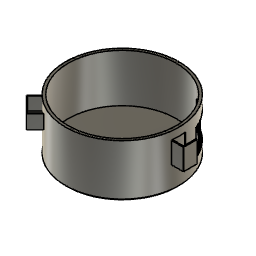
MedWise_shell v1 (Autodesk Fusion 360 design; units mm, degrees)
Autodesk Fusion 360 part; units mm, degrees
sketch "Sketch1" plane through (0, 0, 0) normal (0, 0, 1) x (1, 0, 0)
  circle A0 centre (0, 0) radius 65
  dimension "d1" = 130
  constraint coincident A0.centre origin
  measures "d1" diameter of A0
extrude "Extrude1" add sketch "Sketch1" along normal blind 60
hole "Hole1" at (0, 0, 60) direction (0, 0, -1) diameter 124 depth 55 tip angle 180
ref_plane "WorkPlane1" through (65, 0, 32.9588) normal (1, 0, 0) x (0, -1, 0)
ref_plane "WorkPlane2" through (77.5, 0, 32.9588) normal (1, 0, 0) x (0, -1, 0)
sketch "Sketch2" plane through (77.5, 0, 32.9588) normal (1, 0, 0) x (0, 1, 0)
  line L0 (-8, -8) -> (8, -8)
  line L1 (8, -8) -> (8, 18)
  line L2 (8, 18) -> (-8, 18)
  line L3 (-8, 18) -> (-8, -8)
  line L4 (-8, -8) -> (8, 18) construction
  line L5 (8, -8) -> (-8, 18) construction
  point P0 (0, 5)
  dimension "d9" = 16
  constraint horizontal L0
  constraint perpendicular L0 L1
  constraint parallel L0 L2
  constraint parallel L1 L3
  constraint coincident L4 P0
  constraint coincident L5 P0
  measures "d9" distance of L1.end L2.end
extrude "Extrude2" add sketch "Sketch2" along normal up to surface end surface at (64.677, -6.4719, 40)
extrude "Extrude3" add 1 faces at (77.5, -2.6667, 33.6254) along direction (1, 0, 0) blind 0.5
extrude "Extrude4" cut 1 faces at (73.6667, 0, 24.9588) along direction (0, 0, 1) blind 1
extrude "Extrude5" add 1 faces at (78, -2.6667, 42.6254) along direction (1, 0, 0) blind 0.2
shell "Shell1" thickness 1 removed faces 2 at (69.0705, 8, 34.2921) at (73.8, 0, 50.9588)
ref_plane "WorkPlane3" through (49.7929, 41.7812, 24.979) normal (0.766044, 0.642788, 0) x (0.642788, -0.766044, 0)
sketch "Sketch3" plane through (49.7929, 41.7812, 24.979) normal (0.766044, 0.642788, 0) x (0.642788, -0.766044, 0)
  line L0 (20, -20) -> (-20, -20)
  line L1 (-20, -20) -> (-20, 10)
  line L2 (-20, 10) -> (20, 10)
  line L3 (20, 10) -> (20, -20)
  line L4 (20, -20) -> (-20, 10) construction
  line L5 (-20, -20) -> (20, 10) construction
  point P0 (0, -5)
  dimension "d20" = 40
  constraint horizontal L0
  constraint perpendicular L0 L1
  constraint parallel L0 L2
  constraint parallel L1 L3
  constraint coincident L4 P0
  constraint coincident L5 P0
  measures "d20" distance of L1.end L2.end
extrude "Extrude6" cut sketch "Sketch3" against normal blind 20
fillet "Fillet1" radius 0.4 8 edges at (78.2, 0, 50.9588) (77.7, 8, 50.9588) (78.2, 8, 38.4588) (71.3529, 8, 25.9588) (78.2, 0, 25.9588) (78.2, -8, 38.4588) (71.3529, -8, 50.9588) (71.3529, -8, 25.9588)
fillet "Fillet2" radius 2 1 edges at (-60.6013, -23.505, 0)
ref_plane "WorkPlane4" through (49.7929, 41.7812, 24.979) normal (0.766044, 0.642788, 0) x (0.642788, -0.766044, 0)
ref_plane "WorkPlane5" through (-45.9619, -45.9619, 2.3267) normal (-0.707107, -0.707107, 0) x (-0.707107, 0.707107, 0)
ref_plane "WorkPlane6" through (-55.2958, -55.2958, 2.3267) normal (-0.707107, -0.707107, 0) x (-0.707107, 0.707107, 0)
sketch "Sketch4" plane through (-55.2958, -55.2958, 2.3267) normal (-0.707107, -0.707107, 0) x (-0.707107, 0.707107, 0)
  line L0 (13, -31.7116) -> (-13, -31.7116)
  line L1 (-13, -31.7116) -> (-13, -47.7116)
  line L2 (-13, -47.7116) -> (13, -47.7116)
  line L3 (13, -47.7116) -> (13, -31.7116)
  line L4 (13, -31.7116) -> (-13, -47.7116) construction
  line L5 (-13, -31.7116) -> (13, -47.7116) construction
  point P0 (0, -39.7116)
  dimension "d31" = 26
  dimension "d32" = 16
  constraint horizontal L0
  constraint perpendicular L0 L1
  constraint parallel L0 L2
  constraint parallel L1 L3
  constraint coincident L4 P0
  constraint coincident L5 P0
  measures "d31" distance of L1.end L2.end
  measures "d32" distance of L0.start L2.end
extrude "Extrude7" add sketch "Sketch4" along normal up to surface end surface at (61.9538, 19.6652, 28.9723)
extrude "Extrude8" cut 1 faces at (-52.2316, -58.3599, 39.3716) along direction (0.707107, 0.707107, 0) blind 0.5
shell "Shell2" thickness 1 removed faces 1 at (-52.9418, -50.8867, 50.0383)
